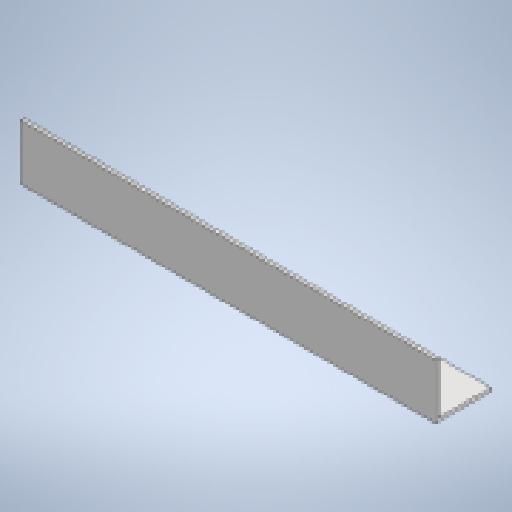
# Autodesk Inventor part: Steel_Angle
Saved by Autodesk Inventor 2023 (Build 270158000, 158)
## iProperties
Created: 2022-04-30
Part Number: Steel_Angle
Material: Generic
Document SubType Name: Modeling
Designer: plebbb
Density: 1 g/cm^3
Appearance: Default
Author: plebbb
Autodesk Inventor part; units mm, degrees
ref_plane "YZ Plane" through (0, 0, 0) normal (1, 0, 0) x (0, 1, 0)
ref_plane "XZ Plane" through (0, 0, 0) normal (0, 1, 0) x (-1, 0, 0)
ref_plane "XY Plane" through (0, 0, 0) normal (0, 0, 1) x (1, 0, 0)
sketch "Sketch1" plane through (0, 0, 0) normal (1, 0, 0) x (0, 1, 0)
  line L0 (50.8, 0) -> (0, 0)
  line L1 (0, 0) -> (0, -50.8)
  line L2 (0, -50.8) -> (3.175, -50.8)
  line L3 (3.175, -50.8) -> (3.175, -3.175)
  line L4 (3.175, -3.175) -> (50.8, -3.175)
  line L5 (50.8, -3.175) -> (50.8, 0)
  dimension "d0" = 50.8
  dimension "d1" = 50.8
  dimension "d2" = 3.175
  constraints: 12 end point, 6 perpendicular, 1 coincident, 1 vertical
  measures "d0" distance of L0.start L0.end
  measures "d1" distance of L0.end L1.end
  measures "d2" distance of L4.end L0.start
extrude "Extrusion1" add sketch "Sketch1" along normal blind 260
body "Solid1"
